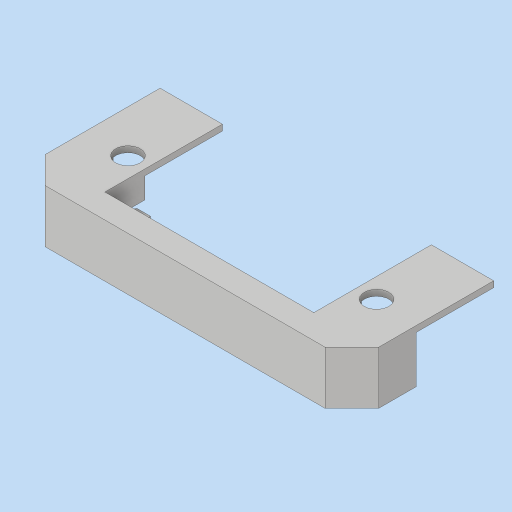
# Autodesk Inventor part: top_DB15
Saved by Autodesk Inventor 2024 (Build 280153000, 153)
## iProperties
Created: 2023-02-28
Part Number: top_DB15
Material: Generic
Document SubType Name: Modeling
Designer: Karbosch
Density: 1 g/cm^3
Appearance: Default
Mass: 1.59007 g
Surface Area: 18.4374 cm^2
Volume: 1.59007 cm^3
Author: Karbosch
Autodesk Inventor part; units mm, degrees
ref_plane "YZ Plane" through (0, 0, 0) normal (1, 0, 0) x (0, 1, 0)
ref_plane "XZ Plane" through (0, 0, 0) normal (0, 1, 0) x (-1, 0, 0)
ref_plane "XY Plane" through (0, 0, 0) normal (0, 0, 1) x (1, 0, 0)
sketch "Sketch2" plane through (0, 0, 0) normal (0, 0, 1) x (1, 0, 0)
  line L0 (0, 0) -> (140, 0)
  line L1 (140, 0) -> (140, 40)
  line L2 (140, 40) -> (0, 40)
  line L3 (0, 40) -> (0, 0)
  dimension "d0" = 140
  dimension "d1" = 40
  constraints: 8 end point, 2 parallel, 1 horizontal, 1 perpendicular
  measures "d0" distance of L2.end L1.end
  measures "d1" distance of L1.end L0.end
extrude "Extrusion1" add sketch "Sketch2" along normal blind 2.4
sketch "Sketch3" plane through (0, 0, 0) normal (0, 0, -1) x (-1, 0, 0)
  line L0 (0, 0) -> (-140, 0) projected
  line L1 (0, 40) -> (0, 0) projected
  line L2 (-140, 40) -> (0, 40) projected
  line L3 (-140, 0) -> (-140, 40) projected
  line L4 (-137.2, 2.8) -> (-2.8, 2.8)
  line L5 (-2.8, 2.8) -> (-2.8, 37.2)
  line L6 (-2.8, 37.2) -> (-137.2, 37.2)
  line L7 (-137.2, 37.2) -> (-137.2, 2.8)
  dimension "d4" = 2.8
  constraints: 8 end point, 3 other
  measures "d4" distance between parallel lines of L0 L4
extrude "Extrusion2" add sketch "Sketch3" against normal blind 20
sketch "Sketch4" plane through (0, 0, 0) normal (0, -1, 0) x (1, 0, 0)
  line L0 (0, 0) -> (140, 0) projected
  circle A0 centre (10.14, 20) radius 1.65
  line L1 (10.14, 20) -> (73.64, 20)
  circle A1 centre (73.64, 20) radius 1.65
  line L2 (12.99, 25.25) -> (70.59, 25.25)
  line L3 (70.59, 25.25) -> (70.59, 13.75)
  line L4 (70.59, 13.75) -> (12.99, 13.75)
  line L5 (12.99, 13.75) -> (12.99, 25.25)
  line L6 (12.99, 25.25) -> (70.59, 13.75) construction
  line L7 (70.59, 25.25) -> (12.99, 13.75) construction
  line L8 (73.64, 20) -> (96.54, 20)
  line L9 (96.54, 20) -> (129.86, 20)
  circle A2 centre (96.54, 20) radius 1.65
  circle A3 centre (129.86, 20) radius 1.65
  line L10 (140, 0) -> (140, 20) projected
  line L11 (99.2, 14.25) -> (127.2, 14.25)
  line L12 (127.2, 14.25) -> (127.2, 25.75)
  line L13 (127.2, 25.75) -> (99.2, 25.75)
  line L14 (99.2, 25.75) -> (99.2, 14.25)
  line L15 (99.2, 14.25) -> (127.2, 25.75) construction
  line L16 (127.2, 14.25) -> (99.2, 25.75) construction
  point P0 (41.79, 19.5)
  point P1 (0, 20)
  point P2 (113.2, 20)
  dimension "d8" = 3.3
  dimension "d9" = 63.5
  dimension "d10" = 3.3
  dimension "d11" = 57.6
  dimension "d12" = 11.5
  dimension "d19" = 22.9
  dimension "d20" = 33.32
  dimension "d21" = 3.3
  dimension "d22" = 3.3
  dimension "d23" = 28
  dimension "d24" = 11.5
  constraints: 30 end point, 5 midpoint, 4 centre point, 4 parallel, 3 coincident, 2 horizontal, 2 perpendicular
  measures "d8" diameter of A0
  measures "d9" distance of L1.start L1.end
  measures "d10" diameter of A1
  measures "d11" distance of L3.end L4.end
  measures "d12" distance of L2.end L3.end
  measures "d19" distance of L8.start L8.end
  measures "d20" distance of L8.end L9.end
  measures "d21" diameter of A2
  measures "d22" diameter of A3
  measures "d23" distance of L13.end L12.end
  measures "d24" distance of L12.end L11.end
extrude "DB37-innern hole" cut sketch "Sketch4" against normal up to surface (2.8 mm away)
sketch "Sketch7" plane through (0, 0, 0) normal (0, -1, 0) x (1, 0, 0)
  arc A0 (8.49, 20) -> (11.79, 20) centre (10.14, 20) ccw projected
  arc A1 (71.99, 20) -> (75.29, 20) centre (73.64, 20) ccw projected
  arc A2 (94.89, 20) -> (98.19, 20) centre (96.54, 20) ccw projected
  arc A3 (128.21, 20) -> (131.51, 20) centre (129.86, 20) ccw projected
  line L0 (10.14, 20) -> (73.64, 20)
  line L1 (96.54, 20) -> (129.86, 20)
  line L2 (6.89, 13.6) -> (76.89, 13.6)
  line L3 (76.89, 13.6) -> (76.89, 20)
  line L4 (76.89, 26.4) -> (6.89, 26.4)
  line L5 (6.89, 20) -> (6.89, 13.6)
  line L6 (6.89, 13.6) -> (76.89, 26.4) construction
  line L7 (76.89, 13.6) -> (6.89, 26.4) construction
  line L8 (93.45, 13.6) -> (132.95, 13.6)
  line L9 (132.95, 13.6) -> (132.95, 20)
  line L10 (132.95, 26.4) -> (93.45, 26.4)
  line L11 (93.45, 20) -> (93.45, 13.6)
  line L12 (93.45, 13.6) -> (132.95, 26.4) construction
  line L13 (132.95, 13.6) -> (93.45, 26.4) construction
  line L14 (79.49, 11) -> (4.29, 11)
  line L15 (4.29, 11) -> (4.29, 20)
  line L16 (79.49, 20) -> (79.49, 11)
  line L17 (8.49, 20) -> (2.8, 20) projected
  line L18 (4.29, 20) -> (6.89, 20)
  line L19 (75.29, 20) -> (94.89, 20) projected
  line L20 (76.89, 20) -> (79.49, 20)
  line L21 (135.55, 11) -> (90.85, 11)
  line L22 (90.85, 11) -> (90.85, 20)
  line L23 (90.85, 29) -> (91.1087, 29)
  line L24 (135.55, 20) -> (135.55, 11)
  line L25 (90.85, 20) -> (93.45, 20)
  line L26 (131.51, 20) -> (140, 20) projected
  line L27 (132.95, 20) -> (135.755, 20)
  point P0 (0, 0)
  point P1 (41.89, 20)
  point P2 (113.2, 20)
  dimension "d25" = 70
  dimension "d26" = 12.8
  dimension "d27" = 39.5
  dimension "d28" = 2.6
  constraints: 50 end point, 9 point on line, 7 midpoint, 7 parallel, 4 perpendicular, 2 horizontal
  measures "d25" distance of L4.end L4.start
  measures "d26" distance of L4.start L2.end
  measures "d27" distance of L10.end L10.start
  measures "d28" distance between parallel lines of L2 L14
extrude "Extrusion4" add sketch "Sketch7" along normal blind 1.5 contours L5 L2 L3 L19 L16 L14 L15 L17 | L11 L8 L9 L26 L24 L21 L22 L19
sketch "Sketch8" plane through (0, -1.5, 0) normal (0, -1, 0) x (1, 0, 0)
  line L0 (6.89, 13.6) -> (6.89, 20) projected
  line L1 (6.89, 20) -> (4.29, 20) projected
  line L2 (4.29, 20) -> (4.29, 11) projected
  line L3 (4.29, 11) -> (79.49, 11) projected
  line L4 (79.49, 11) -> (79.49, 20) projected
  line L5 (79.49, 20) -> (76.89, 20) projected
  line L6 (76.89, 20) -> (76.89, 13.6) projected
  line L7 (76.89, 13.6) -> (6.89, 13.6) projected
  line L8 (93.45, 20) -> (90.85, 20) projected
  line L9 (90.85, 20) -> (90.85, 11) projected
  line L10 (90.85, 11) -> (135.55, 11) projected
  line L11 (135.55, 11) -> (135.55, 20) projected
  line L12 (135.55, 20) -> (132.95, 20) projected
  line L13 (132.95, 20) -> (132.95, 13.6) projected
  line L14 (132.95, 13.6) -> (93.45, 13.6) projected
  line L15 (93.45, 13.6) -> (93.45, 20) projected
  line L16 (79.49, 11) -> (79.49, 20) projected
  line L17 (4.29, 11) -> (79.49, 11)
  line L18 (79.49, 11) -> (79.49, 20)
  line L19 (79.49, 20) -> (75.29, 20)
  line L20 (4.29, 20) -> (4.29, 11)
  line L21 (13.49, 15.1) -> (70.29, 15.1)
  line L22 (70.29, 15.1) -> (70.29, 20)
  line L23 (70.29, 24.9) -> (13.49, 24.9)
  line L24 (13.49, 24.9) -> (13.49, 20)
  line L25 (13.49, 15.1) -> (70.29, 24.9) construction
  line L26 (70.29, 15.1) -> (13.49, 24.9) construction
  line L27 (90.85, 11) -> (135.55, 11)
  line L28 (135.55, 11) -> (135.55, 20)
  line L29 (135.55, 20) -> (131.51, 20)
  line L30 (90.85, 20) -> (90.85, 11)
  line L31 (99.95, 15.1) -> (126.45, 15.1)
  line L32 (126.45, 15.1) -> (126.45, 20)
  line L33 (126.45, 24.9) -> (99.95, 24.9)
  line L34 (99.95, 24.9) -> (99.95, 20)
  line L35 (99.95, 15.1) -> (126.45, 24.9) construction
  line L36 (126.45, 15.1) -> (99.95, 24.9) construction
  line L37 (99.95, 20) -> (99.95, 15.1)
  line L38 (126.45, 20) -> (126.45, 24.9)
  line L39 (99.95, 20) -> (98.19, 20)
  line L40 (126.45, 20) -> (99.95, 20)
  arc A0 (94.89, 20) -> (98.19, 20) centre (96.54, 20) ccw projected
  arc A1 (128.21, 20) -> (131.51, 20) centre (129.86, 20) ccw projected
  arc A2 (71.99, 20) -> (75.29, 20) centre (73.64, 20) ccw projected
  arc A3 (8.49, 20) -> (11.79, 20) centre (10.14, 20) ccw projected
  line L41 (13.49, 20) -> (11.79, 20)
  line L42 (70.29, 20) -> (13.49, 20)
  line L43 (70.29, 20) -> (70.29, 24.9)
  line L44 (13.49, 20) -> (13.49, 15.1)
  line L45 (8.49, 20) -> (4.29, 20)
  line L46 (11.79, 20) -> (8.49, 20)
  line L47 (71.99, 20) -> (70.29, 20)
  line L48 (75.29, 20) -> (71.99, 20)
  line L49 (94.89, 20) -> (90.85, 20)
  line L50 (98.19, 20) -> (94.89, 20)
  line L51 (128.21, 20) -> (126.45, 20)
  line L52 (131.51, 20) -> (128.21, 20)
  point P0 (0, 0)
  point P1 (41.89, 20)
  point P2 (113.2, 20)
  dimension "d31" = 56.8
  dimension "d32" = 9.8
  dimension "d33" = 26.5
  dimension "d34" = 9.8
  constraints: 72 end point, 26 parallel, 8 point on circle, 6 perpendicular, 4 horizontal, 4 midpoint
  measures "d31" distance of L23.end L23.start
  measures "d32" distance of L23.start L21.end
  measures "d33" distance of L33.end L33.start
  measures "d34" distance of L33.start L31.end
extrude "Extrusion5" add sketch "Sketch8" along normal blind 2 contours L7 L6 L5 L4 L3 L2 L1 L0 | L0 L45 A3 L41 L44 L21 L22 L47 A2 L19 L6 L7 | L15 L14 L13 L12 L11 L10 L9 L8 | L49 A0 L39 L37 L31 L32 L51 A1 L29 L13 L14 L15
chamfer "Chamfer1" distance 3.5 angle 45 6 edges at (41.89, 0, 11) (113.2, 0, 11) (79.49, 0, 15.5) (90.85, 0, 15.5) (135.55, 0, 15.5) (4.29, 0, 15.5)
sketch "Sketch9" plane through (0, 0, 2.4) normal (0, 0, 1) x (1, 0, 0)
  line L0 (2.8, 37.2) -> (2.8, 2.8) projected
  line L1 (2.8, 2.8) -> (137.2, 2.8) projected
  line L2 (137.2, 2.8) -> (137.2, 37.2) projected
  line L3 (137.2, 37.2) -> (2.8, 37.2) projected
  line L4 (10, 33) -> (130, 33)
  line L5 (130, 33) -> (130, 7)
  line L6 (130, 7) -> (10, 7)
  line L7 (10, 7) -> (10, 33)
  line L8 (10, 33) -> (130, 7) construction
  line L9 (130, 33) -> (10, 7) construction
  circle A0 centre (130, 33) radius 4
  circle A1 centre (130, 7) radius 4
  circle A2 centre (10, 33) radius 4
  circle A3 centre (10, 7) radius 4
  circle A4 centre (130, 33) radius 2.75
  circle A5 centre (130, 7) radius 2.75
  circle A6 centre (10, 33) radius 2.75
  circle A7 centre (10, 7) radius 2.75
  point P0 (0, 0)
  point P1 (70, 20)
  dimension "d40" = 120
  dimension "d41" = 26
  dimension "d42" = 8
  dimension "d43" = 8
  dimension "d44" = 8
  dimension "d45" = 8
  dimension "d48" = 5.5
  dimension "d49" = 5.5
  dimension "d50" = 5.5
  dimension "d51" = 5.5
  constraints: 12 end point, 8 centre point, 8 coincident, 2 midpoint, 2 parallel, 1 horizontal, 1 perpendicular
  measures "d40" distance of L5.end L6.end
  measures "d41" distance of L4.end L5.end
  measures "d42" diameter of A0
  measures "d43" diameter of A1
  measures "d44" diameter of A2
  measures "d45" diameter of A3
  measures "d48" diameter of A4
  measures "d49" diameter of A5
  measures "d50" diameter of A6
  measures "d51" diameter of A7
extrude "Extrusion6" add sketch "Sketch9" along normal blind 7.6 contours A6 L7 A2 L4 | L4 A2 L7 A6 | A0 L5 A4 L4 | L4 A4 L5 A0 | A3 L6 A7 L7 | L7 A7 L6 A3 | A1 L6 A5 L5 | L5 A5 L6 A1
sketch "Sketch10" plane through (0, 0, 2.4) normal (0, 0, 1) x (1, 0, 0)
  circle A0 centre (10, 33) radius 2.75 projected
  circle A1 centre (10, 7) radius 2.75 projected
  circle A2 centre (130, 33) radius 2.75 projected
  circle A3 centre (130, 7) radius 2.75 projected
  point P0 (0, 0)
hole "Hole1" at (130, 33, 2.4) at (130, 7, 2.4) at (10, 7, 2.4) at (10, 33, 2.4) direction (0, 0, -1) diameter 4.3 end through all
thicken "Thicken1" operation add thickness 2 both sides no extend neighbours no toward (0.9967573, -0.0804666, 0) faces at (13.987, 32.6781, 7.4667)
thicken "Thicken2" operation add thickness 2 both sides no extend neighbours no toward (0.9967573, -0.0804666, 0) faces at (13.987, 6.6781, 7.4667)
thicken "Thicken3" operation add thickness 2 both sides no extend neighbours no toward (0.9967573, -0.0804666, 0) faces at (133.987, 32.6781, 7.4667)
thicken "Thicken4" operation add thickness 2 both sides no extend neighbours no toward (0.9967573, -0.0804666, 0) faces at (133.987, 6.6781, 7.4667)
sketch "Sketch11" plane through (140, 0, 0) normal (1, 0, 0) x (0, 0, -1)
  line L0 (-2.4, 37.2) -> (-2.4, 2.8) projected
  line L1 (-2.4, 37.2) -> (-20, 37.2) projected
  line L2 (-20, 2.8) -> (-20, 37.2) projected
  line L3 (-2.4, 2.8) -> (-20, 2.8) projected
  line L4 (-10, 37.2) -> (-10, 37.2) projected
  line L5 (-10, 30.25) -> (-10, 35.75) projected
  line L6 (0, 0) -> (0, 40) projected
  line L7 (0, 40) -> (-20, 40) projected
  line L8 (-20, 0) -> (-20, 40) projected
  line L9 (0, 0) -> (-20, 0) projected
  line L10 (-20, 2.8) -> (-10, 30.25)
  line L11 (-10, 35.75) -> (-10, 40)
  line L12 (0, 40) -> (-20, 40) projected
  line L13 (-10, 40) -> (-20, 40)
  line L14 (-20, 40) -> (-20, 2.8)
  constraints: 8 end point, 1 collinear, 1 horizontal, 1 midpoint
extrude "Extrusion7" cut sketch "Sketch11" against normal through all contours L11 L5 L10 L2 L1 | L1 L8 L7 L11
chamfer "Chamfer3" distance 4 angle 45 8 edges at (90.85, -3.5, 11) (89.1001, -1.75, 9.2501) (135.55, -3.5, 11) (137.2999, -1.7499, 9.2501) (81.2399, -1.75, 9.2501) (79.49, -3.5, 11) (2.5401, -1.7499, 9.2501) (4.29, -3.5, 11)
mirror "Mirror1" about plane through (70, 20, 20) normal (0, 0, 1) of "Extrusion5", "Extrusion4", "DB37-innern hole", "Extrusion2"
sketch "Sketch12" plane through (0, -3.5, 0) normal (0, -1, 0) x (1, 0, 0)
  line L0 (4.29, 20) -> (4.29, 15.899) projected
  line L1 (4.29, 29) -> (79.49, 29) projected
  line L2 (4.29, 20) -> (79.49, 20)
  line L3 (79.49, 20) -> (79.49, 29)
  line L4 (79.49, 29) -> (4.29, 29)
  line L5 (4.29, 29) -> (4.29, 20)
  line L6 (90.85, 29) -> (135.55, 29) projected
  line L7 (90.85, 20) -> (90.85, 29) projected
  line L8 (135.55, 29) -> (90.85, 29)
  line L9 (90.85, 29) -> (90.85, 20)
  line L10 (90.85, 20) -> (135.55, 20)
  line L11 (135.55, 20) -> (135.55, 29)
  point P0 (0, 0)
  constraints: 16 end point, 4 parallel, 2 horizontal, 2 perpendicular
extrude "Extrusion8" cut sketch "Sketch12" against normal up to surface (6.3 mm away) contours L6 L11 L10 L7 keep common part
sketch "Sketch13" plane through (0, -3.5, 0) normal (0, -1, 0) x (1, 0, 0)
  arc A0 (98.19, 20) -> (94.89, 20) centre (96.54, 20) ccw projected
  arc A1 (131.51, 20) -> (128.21, 20) centre (129.86, 20) ccw projected
  point P0 (0, 0)
hole "Hole2" at (129.86, -3.5, 20) at (96.54, -3.5, 20) direction (0, 1, 0) diameter 7 depth 0.4
sketch "Sketch14" plane through (90.85, 2.8, 29) normal (0, 1, 0) x (1, 0, 0)
  line L0 (0, 9) -> (4.04, 9) projected
  line L1 (0, 0) -> (0, 9) projected
  line L2 (44.7, 0) -> (0, 0) projected
  line L3 (44.7, 9) -> (44.7, 0) projected
  line L4 (40.66, 9) -> (44.7, 9) projected
  arc A0 (37.36, 9) -> (40.66, 9) centre (39.01, 9) ccw projected
  line L5 (36.35, 9) -> (37.36, 9) projected
  line L6 (36.35, 9) -> (36.35, 3.25) projected
  line L7 (36.35, 3.25) -> (8.35, 3.25) projected
  line L8 (8.35, 3.25) -> (8.35, 9) projected
  line L9 (7.34, 9) -> (8.35, 9) projected
  arc A1 (4.04, 9) -> (7.34, 9) centre (5.69, 9) ccw projected
  line L10 (36.35, 9) -> (36.35, 3.25) projected
  line L11 (36.35, 9) -> (36.35, 19)
  line L12 (44.7, 0) -> (44.7, 9) projected
  line L13 (44.7, 9) -> (44.7, 19)
  line L14 (44.7, 19) -> (36.35, 19)
  line L15 (36.35, 3.25) -> (8.35, 3.25) projected
  line L16 (22.35, 3.25) -> (22.35, 7.35)
  line L17 (36.35, 9) -> (36.35, 0)
  line L18 (44.7, 0) -> (0, 0) projected
  line L19 (36.35, 0) -> (44.7, 0)
  line L20 (44.7, 9) -> (44.7, 0)
  circle A2 centre (39.01, 9) radius 1.65
  line L21 (0, 9) -> (0, 0)
  line L22 (4.04, 9) -> (0, 9)
  arc A3 (4.04, 9) -> (7.34, 9) centre (5.69, 9) ccw
  line L23 (8.35, 9) -> (7.34, 9)
  line L24 (8.35, 9) -> (8.35, 3.25)
  line L25 (8.35, 9) -> (8.35, 3.25)
  line L26 (8.35, 9) -> (8.35, 19)
  line L27 (0, 0) -> (0, 9)
  line L28 (0, 9) -> (0, 19)
  line L29 (0, 19) -> (8.35, 19)
  line L30 (8.35, 9) -> (8.35, 0)
  line L31 (8.35, 0) -> (0, 0)
  line L32 (0, 9) -> (0, 0)
  circle A4 centre (5.69, 9) radius 1.65
  point P0 (-90.85, 29)
  dimension "d85" = 10
  constraints: 42 end point, 5 symmetric about line, 4 perpendicular, 4 vertical, 2 coincident, 2 horizontal alignment, 2 point on circle, 1 centre point, 1 midpoint, 1 point on line, 5 other
  measures "d85" distance of L5.start L11.end
extrude "Extrusion9" add sketch "Sketch14" along normal blind 0.8 contours L28 L29 L26 L9 A4 L0 | L0 A1 L9 L8 L30 L2 L1 | L30 L7 L17 L2 | L17 L6 L5 A0 L4 L3 L2 | L4 A2 L5 L11 L14 L13
sketch "Sketch15" plane through (0, -3.5, 0) normal (0, -1, 0) x (1, 0, 0)
  line L0 (135.55, 20) -> (133.36, 20) projected
  line L1 (90.85, 20) -> (90.85, 29) projected
  line L2 (135.55, 20) -> (90.85, 20)
  line L3 (90.85, 20) -> (90.85, 20.4)
  line L4 (90.85, 20.4) -> (135.55, 20.4)
  line L5 (135.55, 20.4) -> (135.55, 20)
  point P0 (0, 0)
  dimension "d88" = 0.4
  constraints: 8 end point, 2 parallel, 1 horizontal, 1 perpendicular, 1 point on line
  measures "d88" distance of L2.end L3.end
extrude "Extrusion10" cut sketch "Sketch15" against normal up to surface (6.3 mm away)
chamfer "Chamfer4" distance 3.6 angle 45 4 edges at (90.85, -0.35, 29) (90.85, 3.2, 29) (135.55, -0.35, 29) (135.55, 3.2, 29)
body "Solid1"
